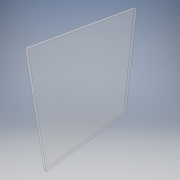
# Autodesk Inventor part: Side Panel
Saved by Autodesk Inventor 2019 (Build 230136000, 136)
## iProperties
Created: 2018-11-13
Part Number: Side Panel
Material: Acrylic, Clear
Document SubType Name: Modeling
Designer: Adhik
Density: 1.19 g/cm^3
Appearance: Transparent - Clear
Author: Adhik
Autodesk Inventor part; units mm, degrees
ref_plane "YZ Plane" through (0, 0, 0) normal (1, 0, 0) x (0, 1, 0)
ref_plane "XZ Plane" through (0, 0, 0) normal (0, 1, 0) x (-1, 0, 0)
ref_plane "XY Plane" through (0, 0, 0) normal (0, 0, 1) x (1, 0, 0)
sketch "Sketch1" plane through (0, 0, 0) normal (1, 0, 0) x (0, 1, 0)
  line L0 (0, -133.35) -> (0, 133.35) construction
  line L1 (-142.24, 0) -> (142.24, 0) construction
  line L2 (101.6, 95.25) -> (-101.6, 95.25)
  line L3 (-101.6, 95.25) -> (-101.6, -95.25)
  line L4 (-101.6, -95.25) -> (101.6, -95.25)
  line L5 (101.6, -95.25) -> (101.6, 95.25)
  point P0 (0, 0)
  point P1 (0, 95.25)
  point P2 (101.6, 0)
  dimension "d0" = 203.2
  dimension "d1" = 190.5
  constraints: 8 end point, 2 midpoint, 2 parallel, 2 point on line, 1 horizontal, 1 perpendicular
  measures "d0" distance of L2.start L2.end
  measures "d1" distance of L4.end L2.start
extrude "Extrusion1" add sketch "Sketch1" along normal blind 5.334
body "Solid1"
